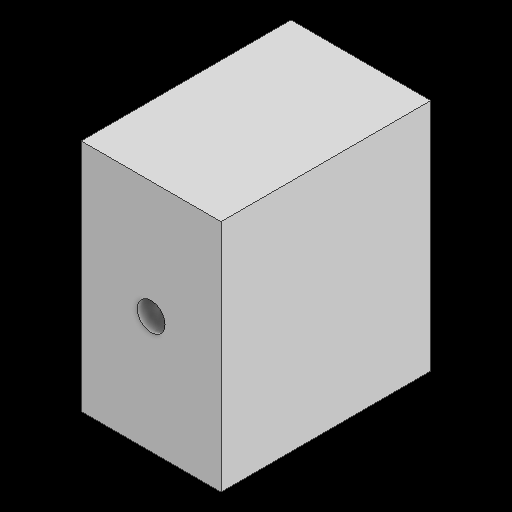
# Autodesk Inventor part: linear_actuator
Saved by Autodesk Inventor 2025.1 (Build 291241000, 241)
## iProperties
Created: 2024-08-22
Part Number: linear_actuator
Material: 일반
Document SubType Name: Modeling
Designer: ojs08
Density: 1 g/cm^3
Appearance: 기본값
Author: ojs08
Autodesk Inventor part; units mm, degrees
ref_plane "YZ Plane" through (0, 0, 0) normal (1, 0, 0) x (0, 1, 0)
ref_plane "XZ Plane" through (0, 0, 0) normal (0, 1, 0) x (-1, 0, 0)
ref_plane "XY Plane" through (0, 0, 0) normal (0, 0, 1) x (1, 0, 0)
sketch "스케치1" plane through (0, 0, 0) normal (0, 0, 1) x (1, 0, 0)
  line L0 (0, 0) -> (20, 0)
  line L1 (20, 0) -> (20, -33.5)
  line L2 (20, -33.5) -> (0, -33.5)
  line L3 (0, -33.5) -> (0, 0)
  dimension "d0" = 33.5
  dimension "d1" = 20
  constraints: 8 end point, 2 parallel, 1 coincident, 1 horizontal, 1 perpendicular
  measures "d0" distance of L2.end L0.start
  measures "d1" distance of L0.start L0.end
extrude "돌출1" add sketch "스케치1" along normal blind 30
sketch "스케치2" plane through (0, 0, 0) normal (0, 0, -1) x (-1, 0, 0)
  circle A0 centre (-10, -16.75) radius 2
  line L0 (0, 0) -> (0, -33.5) projected
  line L1 (-20, 0) -> (0, 0) projected
  dimension "d4" = 4
  dimension "d5" = 10
  dimension "d6" = 16.75
  constraints: 1 centre point
  measures "d4" diameter of A0
  measures "d5" distance from line of L0 A0.centre
  measures "d6" distance from line of L1 A0.centre
extrude "돌출2" cut sketch "스케치2" against normal blind 100
